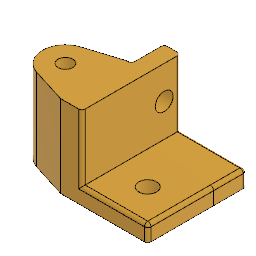
new_bed_bracket v8 (Autodesk Fusion 360 design; units mm, degrees)
Autodesk Fusion 360 part; units mm, degrees
sketch "スケッチ1" plane through (0, 0, 0) normal (0, 0, 1) x (1, 0, 0)
  circle A0 centre (0, 0) radius 2.25
  circle A1 centre (0, 0) radius 7
  line L0 (-2.0936, 6.6796) -> (8.5, 10)
  line L1 (8.5, 10) -> (35, 10)
  line L2 (35, 10) -> (35, -10)
  line L3 (35, -10) -> (8.5, -10)
  line L4 (8.5, -10) -> (-2.0936, -6.6796)
  circle A2 centre (25, 0) radius 2.7
  line L5 (25, 2.7) -> (35, 2.7)
  line L6 (25, -2.7) -> (35, -2.7)
  line L7 (35, 10) -> (10, 10)
  line L8 (10, 10) -> (10, 20)
  line L9 (10, 20) -> (35, 20)
  line L10 (35, 20) -> (35, 10)
  line L11 (10, 20) -> (15, 20)
  line L12 (15, 20) -> (15, 10)
  line L13 (15, 10) -> (10, 10)
  line L14 (10, 10) -> (10, 20)
  line L15 (10, -10) -> (10, 10)
  dimension "d1" = 14
  dimension "d2" = 4.5
  dimension "d3" = 35
  dimension "d4" = 10
  dimension "d5" = 10
  dimension "d6" = 26.5
  dimension "d7" = 26.5
  dimension "d8" = 5.4
  dimension "d9" = 10
  dimension "d36" = 10
  dimension "d37" = 25
  dimension "d38" = 5
  dimension "d47" = 25
  constraint coincident A0.centre A1.centre
  constraint concentric A0 A1
  constraint coincident A1 L0.start
  constraint horizontal L1
  constraint perpendicular L1 L2
  constraint perpendicular L2 L3
  constraint coincident A1 L4.end
  constraint tangent A1 L4
  constraint tangent A1 L0
  constraint coincident A2 L5.start
  constraint coincident L2 L5.end
  constraint perpendicular L2 L5
  constraint coincident A2 L6.start
  constraint coincident L2 L6.end
  constraint perpendicular L2 L6
  constraint tangent A2 L5
  constraint tangent A2 L6
  constraint horizontal A0.centre A2.centre
  constraint horizontal L7
  constraint vertical L8
  constraint horizontal L9
  constraint vertical L10
  constraint horizontal L11
  constraint vertical L12
  constraint horizontal L13
  constraint vertical L14
  constraint coincident L3 L15.start
  constraint coincident L7 L8.start
  constraint perpendicular L3 L15
  measures "d1" diameter of A1
  measures "d2" diameter of A0
  measures "d3" distance of A0.centre L2
  measures "d4" distance of A0.centre L1
  measures "d5" distance of A0.centre L3
  measures "d6" distance of L0.end L2
  measures "d7" distance of L2 L3.end
  measures "d8" diameter of A2
  measures "d9" distance of L2 A2.centre
  measures "d36" distance of L1.end L9.end
  measures "d37" distance of L8.end L9.end
  measures "d38" distance of L12.end L7.end
  measures "d47" distance of L2 L15
extrude "押し出し1" add sketch "スケッチ1" against normal blind 5 contours A1 | A1 L0 L1 L3 L4 L15 | L1 L2 L3 A2 L5 L6 L7 L13 L15 | L2 A2 L5 L6
sketch "スケッチ2" plane through (0, 0, 0) normal (0, 0, 1) x (1, 0, 0)
  line L0 (8.5, 10) -> (35, 10)
  line L1 (35, -10) -> (8.5, -10)
  line L2 (15, 10) -> (15, -10)
  line L3 (8.5, 10) -> (8.5, -10)
  line L4 (10, 10) -> (10, -10)
  line L5 (8.5, 5) -> (10, 5)
  line L6 (8.5, -5) -> (10, -5)
  dimension "d12" = 1.5
  dimension "d13" = 5
  dimension "d14" = 5
  dimension "d15" = 5
  constraint coincident L0 L2.start
  constraint coincident L1 L2.end
  constraint perpendicular L1 L2
  constraint coincident L0.start L3.start
  constraint coincident L1.end L3.end
  constraint coincident L0 L4.start
  constraint coincident L1 L4.end
  constraint perpendicular L1 L4
  constraint coincident L4 L5.end
  constraint perpendicular L4 L5
  constraint coincident L3 L6.start
  constraint coincident L4 L6.end
  constraint perpendicular L4 L6
  measures "d12" distance of L3 L4
  measures "d13" distance of L2 L4
  measures "d14" distance of L0 L5
  measures "d15" distance of L1 L6
extrude "押し出し2" add sketch "スケッチ2" along normal blind 20 contours L0 L1 L2 L4
extrude "Extrude6" add sketch "スケッチ1" along normal up to surface (20 mm away) contours A1 | A1 L0 L1 L3 L4 L15
fillet "フィレット1" radius 1 2 edges at (15, -10, 10) (35, -10, -2.5)
extrude "Extrude3" add sketch "スケッチ1" against normal blind 5 contours L1 L7 L8 L9 L11 L12 L13 L14 | L1 L7 L9 L10 L12
extrude "Extrude4" add sketch "スケッチ1" along normal up to surface (20 mm away) contours L1 L7 L8 L9 L11 L12 L13 L14
sketch "Sketch3" plane through (10, 0, 0) normal (-1, 0, 0) x (0, -1, 0)
  line L0 (-20, 20) -> (-20, -5)
  line L1 (-20, -5) -> (-10, -5)
  line L2 (-10, -5) -> (-10, 20)
  line L3 (-10, 20) -> (-20, 20)
  line L4 (-10, 0) -> (-20, 0) construction
  line L5 (-15, 0) -> (-15, 20) construction
  line L6 (-20, 0) -> (-20, 20) construction
  line L7 (-20, 10) -> (-10, 10) construction
  circle A0 centre (-15, 10) radius 2.7
  dimension "d43" = 5.4
  constraint midpoint L4 L5.start
  constraint midpoint L3 L5.end
  constraint midpoint L6 L7.start
  constraint coincident L2 L7.end
  constraint midpoint L7 A0.centre
  measures "d43" diameter of A0
extrude "Extrude5" cut sketch "Sketch3" against normal blind 5 contours A0
fillet "Fillet7" radius 1 8 edges at (15, 20, 10) (10, 20, 7.5) (35, 0.5, 0) (35, 15, 0) (34.7071, -9.7071, 0) (24, -10, 0) (25, 20, 0) (35, 20, -2.5)
fillet "Fillet9" radius 1 1 edges at (10, 10, 7.5)
equation "d3 = 29 mm + 6 mm"
equation "d6 = 20.5 mm + 6 mm"
equation "d7 = 20.5 mm + 6 mm"
equation "d9 = 4 mm + 6 mm"
